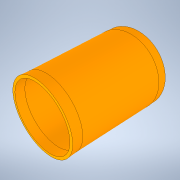
# Autodesk Inventor part: Конусный барабан катушки
Saved by Autodesk Inventor 2021.1 (Build 251245010, 245A)
## iProperties
Created: 2026-04-13
Part Number: Конусный барабан катушки
Material: Типовые
Document SubType Name: Modeling
Designer: Андрей Тарасов
Density: 1 g/cm^3
Appearance: По умолчанию
Author: Андрей Тарасов
Autodesk Inventor part; units mm, degrees
ref_plane "YZ Plane" through (0, 0, 0) normal (1, 0, 0) x (0, 1, 0)
ref_plane "XZ Plane" through (0, 0, 0) normal (0, 1, 0) x (-1, 0, 0)
ref_plane "XY Plane" through (0, 0, 0) normal (0, 0, 1) x (1, 0, 0)
sketch "Эскиз4" plane through (0, 0, 0) normal (0, 1, 0) x (-1, 0, 0)
  line L0 (20.7, 60) -> (23.2, 6)
  line L1 (25, 6) -> (22.5, 60)
  line L2 (0, -13.2) -> (0, 79.2) construction
  line L3 (25, 6) -> (23.2, 6) construction
  line L4 (23.2, 6) -> (23.2, 0)
  line L5 (23.2, 0) -> (25, 0)
  line L6 (25, 0) -> (25, 6)
  line L7 (22.5, 60) -> (20.7, 60) construction
  line L8 (20.7, 60) -> (20.7, 66)
  line L9 (20.7, 66) -> (22.5, 66)
  line L10 (22.5, 66) -> (22.5, 60)
  line L11 (25.86, 0) -> (19.84, 0) construction
  dimension "d11" = 25
  dimension "d13" = 22.5
  dimension "d16" = 6
  dimension "d17" = 1.8
  dimension "d18" = 66
  constraints: 20 end point, 6 parallel, 3 horizontal, 2 perpendicular, 1 other
  measures "d11" distance from line of L1.start L2
  measures "d13" distance from line of L2 L1.end
  measures "d16" distance between parallel lines of L7 L9
  measures "d17" distance between parallel lines of L4 L6
  measures "d18" distance between parallel lines of L5 L9
revolve "Вращение1" add sketch "Эскиз4" angle 360 about axis through (0, 0, -10) along (0, 0, 1)
